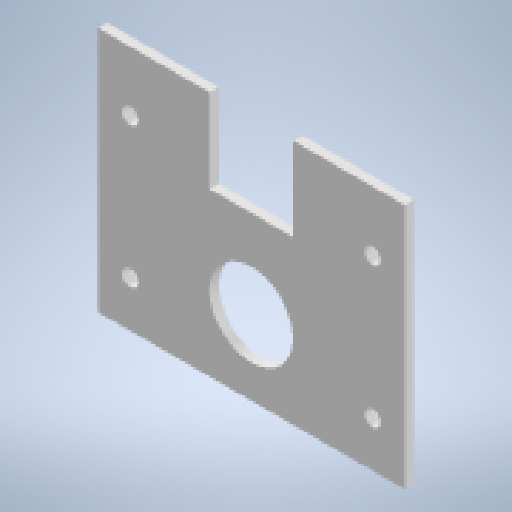
# Autodesk Inventor part: DIFF_PLATE_ROD_SHORT
Saved by Autodesk Inventor 2025.1 (Build 291241000, 241)
## iProperties
Created: 2024-01-10
Part Number: DIFF_PLATE_ROD_SHORT
Material: Generic
Document SubType Name: Modeling
Designer: bugme
Density: 1 g/cm^3
Appearance: Default
Author: bugme
Autodesk Inventor part; units mm, degrees
ref_plane "YZ Plane" through (0, 0, 0) normal (1, 0, 0) x (0, 1, 0)
ref_plane "XZ Plane" through (0, 0, 0) normal (0, 1, 0) x (-1, 0, 0)
ref_plane "XY Plane" through (0, 0, 0) normal (0, 0, 1) x (1, 0, 0)
sketch "Sketch1" plane through (0, 0, 0) normal (0, 0, 1) x (1, 0, 0)
  line L0 (0, -61.7474) -> (0, 56.6674) projected
  line L1 (52.705, 39.751) -> (52.705, -44.831)
  line L2 (52.705, -44.831) -> (-52.705, -44.831)
  line L3 (-52.705, -44.831) -> (-52.705, 39.751)
  line L4 (-73.787, 0) -> (73.787, 0) projected
  line L5 (-14.351, 39.751) -> (-14.351, 11.049)
  line L6 (-14.351, 11.049) -> (14.351, 11.049)
  line L7 (14.351, 11.049) -> (14.351, 39.751)
  line L8 (-52.705, 39.751) -> (-14.351, 39.751)
  line L9 (14.351, 39.751) -> (52.705, 39.751)
  line L10 (0, -44.831) -> (0, -19.177)
  circle A0 centre (0, -19.177) radius 14.2875
  point P0 (0, 0)
  dimension "d0" = 105.41
  dimension "d1" = 84.582
  dimension "d2" = 28.702
  dimension "d3" = 28.702
  dimension "d4" = 25.654
  dimension "d5" = 28.575
  constraints: 18 end point, 4 perpendicular, 2 horizontal, 2 vertical, 1 centre point, 1 coincident, 1 midpoint, 1 point on line, 1 symmetric about line, 1 other
  measures "d0" distance of L3.end L1.start
  measures "d1" distance of L1.start L1.end
  measures "d2" distance of L5.start L5.end
  measures "d3" distance of L5.end L6.end
  measures "d4" distance of L10.start L10.end
  measures "d5" diameter of A0
extrude "Extrusion1" add sketch "Sketch1" along normal blind 3.175 contours L2 L3 L4 L0 A0 | L0 A0 L4 L1 L2 | L4 L0 L6 L7 L9 L1 | L3 L8 L5 L6 L0 L4
sketch "Sketch2" plane through (0, 0, 3.175) normal (0, 0, 1) x (1, 0, 0)
  line L0 (52.705, -44.831) -> (52.705, 39.751) projected
  line L1 (-52.705, -44.831) -> (52.705, -44.831) projected
  point P0 (0, 0)
  point P1 (41.656, 19.177)
  point P2 (41.656, -29.083)
  dimension "d15" = 48.26
  dimension "d16" = 11.049
  dimension "d17" = 11.049
  dimension "d18" = 15.748
  measures "d15" distance of point (41.656, -29.083) point (41.656, 19.177)
  measures "d16" distance from line of L0 point (41.656, 19.177)
  measures "d17" distance from line of L0 point (41.656, -29.083)
  measures "d18" distance from line of L1 point (41.656, -29.083)
hole "Hole1" at (41.656, 19.177, 3.175) at (41.656, -29.083, 3.175) direction (0, 0, -1) diameter 5.5118 end through all clearance for "Flat Head Machine Screw" size "M5" standard "Ansi Metric M Profile"
mirror "Mirror1" about plane through (0, 0, 0) normal (1, 0, 0) of "Hole1"
body "Solid1"
